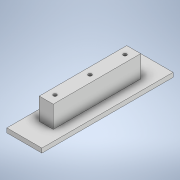
# Autodesk Inventor part: Pin holder
Saved by Autodesk Inventor 2022 (Build 260153000, 153)
## iProperties
Created: 2022-03-17
Part Number: Pin holder
Material: Generic
Document SubType Name: Modeling
Designer: Alexa
Density: 1 g/cm^3
Appearance: Default
Author: Alexa
Autodesk Inventor part; units mm, degrees
ref_plane "YZ Plane" through (0, 0, 0) normal (1, 0, 0) x (0, 1, 0)
ref_plane "XZ Plane" through (0, 0, 0) normal (0, 1, 0) x (-1, 0, 0)
ref_plane "XY Plane" through (0, 0, 0) normal (0, 0, 1) x (1, 0, 0)
sketch "Sketch1" plane through (0, 0, 0) normal (0, 1, 0) x (-1, 0, 0)
  line L0 (0, 0) -> (40, 0)
  line L1 (40, 0) -> (40, -150)
  line L2 (40, -150) -> (0, -150)
  line L3 (0, -150) -> (0, 0)
  dimension "d0" = 40
  dimension "d1" = 150
  constraints: 8 end point, 2 parallel, 1 horizontal, 1 perpendicular
  measures "d0" distance of L1.end L2.end
  measures "d1" distance of L0.end L1.end
extrude "Extrusion1" add sketch "Sketch1" along normal blind 5
sketch "Sketch2" plane through (0, 5, 0) normal (0, 1, 0) x (1, 0, 0)
  line L0 (-40, 0) -> (0, 0) projected
  line L1 (0, 150) -> (-40, 150) projected
  line L2 (-40, 0) -> (-20, 0)
  line L3 (-20, 0) -> (-20, 150)
  line L4 (-20, 150) -> (-40, 150)
  line L5 (-40, 150) -> (-40, 0)
  line L6 (-20, 0) -> (-20, 75)
  line L7 (-20, 75) -> (-20, 35)
  line L8 (-20, 35) -> (-28, 35)
  line L9 (-28, 35) -> (-28, 25)
  line L10 (-28, 25) -> (-20, 25)
  line L11 (-20, 25) -> (-20, 35)
  line L12 (-20, 25) -> (-12, 25)
  line L13 (-12, 25) -> (-12, 35)
  line L14 (-12, 35) -> (-20, 35)
  line L15 (-20, 35) -> (-20, 25)
  line L16 (-20, 75) -> (-20, 115)
  line L17 (-20, 115) -> (-28, 115)
  line L18 (-28, 115) -> (-28, 125)
  line L19 (-28, 125) -> (-20, 125)
  line L20 (-20, 125) -> (-20, 115)
  line L21 (-20, 115) -> (-12, 115)
  line L22 (-12, 115) -> (-12, 125)
  line L23 (-12, 125) -> (-20, 125)
  line L24 (-20, 125) -> (-20, 115)
  line L25 (-28, 125) -> (-12, 125)
  line L26 (-12, 125) -> (-12, 25)
  line L27 (-12, 25) -> (-28, 25)
  line L28 (-28, 25) -> (-28, 125)
  dimension "d4" = 75
  dimension "d5" = 40
  dimension "d6" = 8
  dimension "d7" = 10
  dimension "d8" = 8
  dimension "d9" = 40
  dimension "d10" = 10
  constraints: 54 end point, 12 parallel, 6 horizontal, 6 perpendicular, 4 point on line, 2 midpoint
  measures "d4" distance of L2.end L6.end
  measures "d5" distance of L6.end L7.end
  measures "d6" distance of L10.end L9.end
  measures "d7" distance of L9.end L8.end
  measures "d8" distance of L14.end L13.end
  measures "d9" distance of L6.end L16.end
  measures "d10" distance of L17.end L18.end
extrude "Extrusion2" add sketch "Sketch2" along normal blind 25 contours L10 L9 L8 L3 | L3 L14 L13 L12 | L8 L28 L17 L3 | L3 L21 L26 L14 | L23 L22 L21 L3 | L3 L17 L18 L19
sketch "Sketch3" plane through (0, 30, 0) normal (0, 1, 0) x (1, 0, 0)
  line L0 (-12, 25) -> (-28, 25) projected
  line L1 (-20, 25) -> (-20, 125)
  line L2 (-12, 125) -> (-28, 125) projected
  line L3 (-20, 25) -> (-20, 75)
  line L4 (-20, 75) -> (-20, 35)
  line L5 (-20, 35) -> (-20, 115)
  circle A0 centre (-20, 35) radius 2
  circle A1 centre (-20, 75) radius 2
  circle A2 centre (-20, 115) radius 2
  point P0 (0, 0)
  dimension "d13" = 40
  dimension "d14" = 80
  dimension "d15" = 4
  dimension "d16" = 4
  dimension "d17" = 4
  constraints: 8 end point, 3 centre point, 3 coincident, 3 midpoint, 2 point on line
  measures "d13" distance of L3.end L4.end
  measures "d14" distance of L4.end L5.end
  measures "d15" diameter of A0
  measures "d16" diameter of A1
  measures "d17" diameter of A2
extrude "Extrusion3" cut sketch "Sketch3" against normal blind 12.5
body "Solid1"
